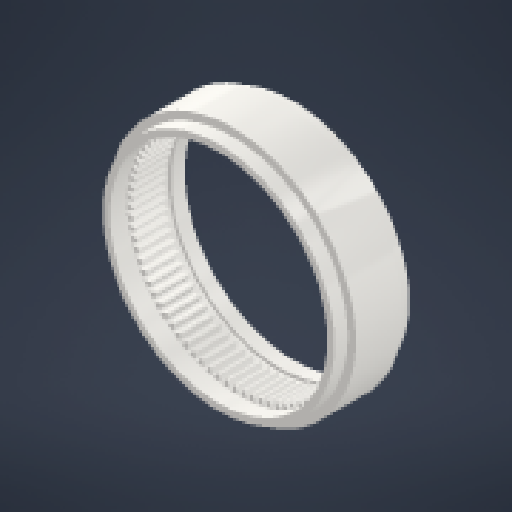
# Autodesk Inventor part: Spur Gear1
Saved by Autodesk Inventor 2024.2 (Build 282272000, 272)
## iProperties
CustomPartVersion: 1
Created: 2026-01-16
Part Number: Spur Gear1
Material: Steel
Document SubType Name: Modeling
Designer: 4aida
Categories: <?xml version="1.0" encoding="UTF-16"?> <MemberInstance><Categories><FamilyTemplate><FamilyTemplateParameter ValueType="xs:double" Id="1" ObjectReferenceKey="da_z" ObjectType="kUserParameterObject"/><FamilyTemplateParameter ValueType="xs:double" Id="2" ObjectReferenceKey="da_b" ObjectType="kUserParameterObject"/><FamilyTemplateParameter ValueType="xs:double" Id="3" ObjectReferenceKey="da_beta" ObjectType="kUserParameterObject"/><FamilyTemplateParameter ValueType="xs:double" Id="4" ObjectReferenceKey="da_da" ObjectType="kUserParameterObject"/><FamilyTemplateParameter ValueType="xs:double" Id="5" ObjectReferenceKey="da_aw" ObjectType="kUserParameterObject"/><FamilyTemplateParameter ValueType="xs:string" Id="6" ObjectReferenceKey="EAIAABAAAACIAQAAAAAAAIAAAAAAAAAA" ObjectType="83910656" SubObjectId="SurfaceGeometry"/></FamilyTemplate><ParamToTemplateMap><ParamToTemplate CategoryParameter="//CategoryParameter[@InternalName='046C89C9-8512-4d59-83FE-43B91F4F132A']" TemplateParameter="1"/><ParamToTemplate CategoryParameter="//CategoryParameter[@InternalName='2552DF32-E462-4b46-AEBF-C6C7768E72AC']" TemplateParameter="2"/><ParamToTemplate CategoryParameter="//CategoryParameter[@InternalName='C9EE641D-15FC-4fae-A226-E94C4372FDD7']" TemplateParameter="3"/><ParamToTemplate><ParamToTemplate CategoryParameter="//CategoryParameter[@InternalName='00B6519A-459B-49c7-AD84-2E56D39A5744']" ConstantValue="0.000000"/></ParamToTemplate><ParamToTemplate><ParamToTemplate CategoryParameter="//CategoryParameter[@InternalName='04B31F0E-C7A6-4894-AA32-9629BEFACF47']" ConstantValue="1.000000"/></ParamToTemplate><ParamToTemplate><ParamToTemplate CategoryParameter="//CategoryParameter[@InternalName='43CBEC2E-7847-49e7-A936-2F7889FCB2D9']" ConstantValue="0.250000"/></ParamToTemplate><ParamToTemplate><ParamToTemplate CategoryParameter="//CategoryParameter[@InternalName='B1EFC894-105D-4ebd-86BF-FA20ED196853']" ConstantValue="0.350000"/></ParamToTemplate><ParamToTemplate><ParamToTemplate CategoryParameter="//CategoryParameter[@InternalName='51175063-3D10-4879-93E8-6246FE8B403D']" ConstantValue="2060000000.000000"/></ParamToTemplate><ParamToTemplate><ParamToTemplate CategoryParameter="//CategoryParameter[@InternalName='A3A52E27-4454-46a9-B0BD-C932399B70AF']" ConstantValue="0.300000"/></ParamToTemplate><ParamToTemplate><ParamToTemplate CategoryParameter="//CategoryParameter[@InternalName='91B76062-C214-41d9-B1B9-14D2AB99603D']" ConstantValue="0.080000"/></ParamToTemplate><ParamToTemplate><ParamToTemplate CategoryParameter="//CategoryParameter[@InternalName='374E806E-8B8A-4dda-A9AA-1039D6500AD2']" ConstantValue="12.500000"/></ParamToTemplate><ParamToTemplate><ParamToTemplate CategoryParameter="//CategoryParameter[@InternalName='2D373A89-B862-43d6-8D0B-0CBF12AB9F6C']" ConstantValue="0.349066"/></ParamToTemplate><ParamToTemplate CategoryParameter="//CategoryParameter[@InternalName='37777632-D6A2-4fac-9D53-DB8ACD95C989']" TemplateParameter="4"/><ParamToTemplate CategoryParameter="//CategoryParameter[@InternalName='FD1017F1-B727-4f7e-9707-0F86F1FF9423']" TemplateParameter="5"/><ParamToTemplate><ParamToTemplate CategoryParameter="//CategoryParameter[@InternalName='9E1B4470-B2D3-4ff1-B813-535BB4CDF51A']" ConstantValue="3520000.000000"/></ParamToTemplate><ParamToTemplate><ParamToTemplate CategoryParameter="//CategoryParameter[@InternalName='F8452263-BFF6-458c-9FB1-07C4B99E95CD']" ConstantValue="11400000.000000"/></ParamToTemplate><ParamToTemplate><ParamToTemplate CategoryParameter="//CategoryParameter[@InternalName='3E3BB259-FD49-497f-8171-6EBC954A3479']" ConstantValue="2.000000"/></ParamToTemplate><ParamToTemplate CategoryParameter="//CategoryParameter[@InternalName='27C3BAF2-7550-4e4b-AE2C-0DB134B7D9B7']" TemplateParameter="6"/></ParamToTemplateMap><Category DisplayName="Gear" InternalName="DC85795E-93AB-48d5-8EEE-5A27447B64BD" Mnemonic="Gear"><CategoryParameter DisplayName="z" InternalName="046C89C9-8512-4d59-83FE-43B91F4F132A" Mnemonic="z"/><CategoryParameter DisplayName="b" InternalName="2552DF32-E462-4b46-AEBF-C6C7768E72AC" Mnemonic="b"/><CategoryParameter DisplayName="||b|" InternalName="C9EE641D-15FC-4fae-A226-E94C4372FDD7" Mnemonic="beta"/><CategoryParameter DisplayName="x" InternalName="00B6519A-459B-49c7-AD84-2E56D39A5744" Mnemonic="x"/><CategoryParameter DisplayName="a*" InternalName="04B31F0E-C7A6-4894-AA32-9629BEFACF47" Mnemonic="a"/><CategoryParameter DisplayName="c*" InternalName="43CBEC2E-7847-49e7-A936-2F7889FCB2D9" Mnemonic="c"/><CategoryParameter DisplayName="r|.f|*" InternalName="B1EFC894-105D-4ebd-86BF-FA20ED196853" Mnemonic="rf"/><CategoryParameter DisplayName="E" InternalName="51175063-3D10-4879-93E8-6246FE8B403D" Mnemonic="E"/><CategoryParameter DisplayName="||m|" InternalName="A3A52E27-4454-46a9-B0BD-C932399B70AF" Mnemonic="mi"/><Category DisplayName="SpurGear" InternalName="26C5A22E-A91E-4dfd-A3B3-23CCAFAE1764" Mnemonic="SpurGear"><CategoryParameter DisplayName="m" InternalName="91B76062-C214-41d9-B1B9-14D2AB99603D" Mnemonic="m"/><CategoryParameter DisplayName="P" InternalName="374E806E-8B8A-4dda-A9AA-1039D6500AD2" Mnemonic="PP"/><CategoryParameter DisplayName="||a|" InternalName="2D373A89-B862-43d6-8D0B-0CBF12AB9F6C" Mnemonic="alpha"/><CategoryParameter DisplayName="d|.a|" InternalName="37777632-D6A2-4fac-9D53-DB8ACD95C989" Mnemonic="da"/><CategoryParameter DisplayName="a|.w|" InternalName="FD1017F1-B727-4f7e-9707-0F86F1FF9423" Mnemonic="aw"/><CategoryParameter DisplayName="||s||.Flim|" InternalName="9E1B4470-B2D3-4ff1-B813-535BB4CDF51A" Mnemonic="sFlim"/><CategoryParameter DisplayName="||s||.Hlim|" InternalName="F8452263-BFF6-458c-9FB1-07C4B99E95CD" Mnemonic="sHlim"/><CategoryParameter DisplayName="type" InternalName="3E3BB259-FD49-497f-8171-6EBC954A3479" Mnemonic="type"/><Category DisplayName="InternalSpurGear" InternalName="7CF704F6-14A9-42f8-93CE-E71DF57C2B55" Mnemonic="InternalSpurGear"><CategoryParameter DisplayName="PitchDiameter" InternalName="27C3BAF2-7550-4e4b-AE2C-0DB134B7D9B7" Mnemonic="IDS_PITCHDIAM"/></Category></Category></Category></Categories></MemberInstance>
Density: 1 g/cm^3
Appearance: Steel
Author: 4aida
Autodesk Inventor part; units mm, degrees
sketch "Sketch1" plane through (0, 0, 0) normal (0, 0, 1) x (1, 0, 0)
  circle A0 centre (0, 0) radius 36.3
  dimension "d0" = 72.6
  constraints: 1 centre point
  measures "d0" diameter of A0
extrude "Extrusion1" add sketch "Sketch1" along normal mid plane 10
ref_plane "Work Plane2" through (0, 0, 0) normal (0, 0, 1) x (1, 0, 0)
sketch "Sketch2" plane through (0, 0, -5) normal (0, 0, -1) x (-1, 0, 0)
  circle A0 centre (0, 0) radius 36.3 projected
  circle A1 centre (0, 0) radius 32
  dimension "d3" = 64
  constraints: 1 centre point, 1 coincident
  measures "d3" diameter of A1
surface extrude "Pitch Diameter" sketch "Sketch2" against normal through all shown no curves A1
ref_plane "Work Plane8" through (0, 0, 0) normal (0.999229, 0.0392598, 0) x (0, 0, 1)
ref_plane "Work Plane9" through (0, 0, 0) normal (1, 0, 0) x (0, 1, 0)
spur gear teeth "Spur Gear" teeth 80 pitch diameter 64 tip diameter 62.4 root diameter 66 face width 10 start plane through (0, 0, -5) normal (0, 0, -1) x (-1, 0, 0)
sketch "Sketch3" plane through (0, 0, 5) normal (0, 0, 1) x (1, 0, 0)
  arc A0 (2.912, -32.8713) -> (3.3628, -31.0182) centre (-7.2848, -29.4092) ccw projected
  arc A1 (2.2661, -32.9221) -> (2.912, -32.8713) centre (0, 0) ccw projected
  arc A2 (1.5309, -31.1624) -> (2.2661, -32.9221) centre (11.7957, -27.9075) ccw projected
  arc A3 (0.9188, -31.1865) -> (1.5309, -31.1624) centre (0, 0) ccw projected
  arc A4 (0.324, -32.9984) -> (0.9188, -31.1865) centre (-9.5697, -28.747) ccw projected
  arc A5 (-0.324, -32.9984) -> (0.324, -32.9984) centre (0, 0) ccw projected
  arc A6 (-0.9188, -31.1865) -> (-0.324, -32.9984) centre (9.5697, -28.747) ccw projected
  arc A7 (-1.5309, -31.1624) -> (-0.9188, -31.1865) centre (0, 0) ccw projected
  arc A8 (-2.2661, -32.9221) -> (-1.5309, -31.1624) centre (-11.7957, -27.9075) ccw projected
  arc A9 (-2.912, -32.8713) -> (-2.2661, -32.9221) centre (0, 0) ccw projected
  arc A10 (-3.3628, -31.0182) -> (-2.912, -32.8713) centre (7.2848, -29.4092) ccw projected
  arc A11 (-3.9712, -30.9462) -> (-3.3628, -31.0182) centre (0, 0) ccw projected
  arc A12 (-4.8421, -32.6428) -> (-3.9712, -30.9462) centre (-13.9489, -26.896) ccw projected
  arc A13 (-5.4821, -32.5415) -> (-4.8421, -32.6428) centre (0, 0) ccw projected
  arc A14 (-5.7861, -30.6588) -> (-5.4821, -32.5415) centre (4.9549, -29.8901) ccw projected
  arc A15 (-6.3869, -30.5393) -> (-5.7861, -30.6588) centre (0, 0) ccw projected
  arc A16 (-7.3883, -32.1623) -> (-6.3869, -30.5393) centre (-16.0162, -25.7187) ccw projected
  arc A17 (-8.0183, -32.011) -> (-7.3883, -32.1623) centre (0, 0) ccw projected
  arc A18 (-8.1737, -30.1103) -> (-8.0183, -32.011) centre (2.5945, -30.1867) ccw projected
  arc A19 (-8.7633, -29.944) -> (-8.1737, -30.1103) centre (0, 0) ccw projected
  arc A20 (-9.889, -31.4835) -> (-8.7633, -29.944) centre (-17.9847, -24.3828) ccw projected
  arc A21 (-10.5052, -31.2832) -> (-9.889, -31.4835) centre (0, 0) ccw projected
  arc A22 (-10.511, -29.3762) -> (-10.5052, -31.2832) centre (0.218, -30.2972) ccw projected
  arc A23 (-11.0857, -29.1641) -> (-10.511, -29.3762) centre (0, 0) ccw projected
  arc A24 (-12.3286, -30.6105) -> (-11.0857, -29.1641) centre (-19.8423, -22.8966) ccw projected
  arc A25 (-12.9273, -30.3626) -> (-12.3286, -30.6105) centre (0, 0) ccw projected
  arc A26 (-12.7834, -28.4609) -> (-12.9273, -30.3626) centre (-2.1597, -30.2209) ccw projected
  arc A27 (-13.3397, -28.2045) -> (-12.7834, -28.4609) centre (0, 0) ccw projected
  arc A28 (-14.6923, -29.5489) -> (-13.3397, -28.2045) centre (-21.5775, -21.2692) ccw projected
  arc A29 (-15.2696, -29.2547) -> (-14.6923, -29.5489) centre (0, 0) ccw projected
  arc A30 (-14.977, -27.3702) -> (-15.2696, -29.2547) centre (-4.5242, -29.9583) ccw projected
  arc A31 (-15.5115, -27.0709) -> (-14.977, -27.3702) centre (0, 0) ccw projected
  arc A32 (-16.9654, -28.305) -> (-15.5115, -27.0709) centre (-23.1798, -19.5107) ccw projected
  arc A33 (-17.5179, -27.9665) -> (-16.9654, -28.305) centre (0, 0) ccw projected
  arc A34 (-17.0783, -26.1108) -> (-17.5179, -27.9665) centre (-6.8607, -29.511) ccw projected
  arc A35 (-17.5876, -25.7704) -> (-17.0783, -26.1108) centre (0, 0) ccw projected
  arc A36 (-19.1339, -26.8867) -> (-17.5876, -25.7704) centre (-24.6391, -17.6318) ccw projected
  arc A37 (-19.6581, -26.5058) -> (-19.1339, -26.8867) centre (0, 0) ccw projected
  arc A38 (-19.0743, -24.6903) -> (-19.6581, -26.5058) centre (-9.155, -28.8817) ccw projected
  arc A39 (-19.5553, -24.3111) -> (-19.0743, -24.6903) centre (0, 0) ccw projected
  arc A40 (-21.1844, -25.3026) -> (-19.5553, -24.3111) centre (-25.9465, -15.6443) ccw projected
  arc A41 (-21.6771, -24.8818) -> (-21.1844, -25.3026) centre (0, 0) ccw projected
  arc A42 (-20.9526, -23.1177) -> (-21.6771, -24.8818) centre (-11.3928, -28.0744) ccw projected
  arc A43 (-21.4025, -22.7018) -> (-20.9526, -23.1177) centre (0, 0) ccw projected
  arc A44 (-23.1043, -23.5625) -> (-21.4025, -22.7018) centre (-27.094, -13.5604) ccw projected
  arc A45 (-23.5625, -23.1043) -> (-23.1043, -23.5625) centre (0, 0) ccw projected
  arc A46 (-22.7018, -21.4025) -> (-23.5625, -23.1043) centre (-13.5604, -27.094) ccw projected
  arc A47 (-23.1177, -20.9526) -> (-22.7018, -21.4025) centre (0, 0) ccw projected
  arc A48 (-24.8818, -21.6771) -> (-23.1177, -20.9526) centre (-28.0744, -11.3928) ccw projected
  arc A49 (-25.3026, -21.1844) -> (-24.8818, -21.6771) centre (0, 0) ccw projected
  arc A50 (-24.3111, -19.5553) -> (-25.3026, -21.1844) centre (-15.6443, -25.9465) ccw projected
  arc A51 (-24.6903, -19.0743) -> (-24.3111, -19.5553) centre (0, 0) ccw projected
  arc A52 (-26.5058, -19.6581) -> (-24.6903, -19.0743) centre (-28.8817, -9.155) ccw projected
  arc A53 (-26.8867, -19.1339) -> (-26.5058, -19.6581) centre (0, 0) ccw projected
  arc A54 (-25.7704, -17.5876) -> (-26.8867, -19.1339) centre (-17.6318, -24.6391) ccw projected
  arc A55 (-26.1108, -17.0783) -> (-25.7704, -17.5876) centre (0, 0) ccw projected
  arc A56 (-27.9665, -17.5179) -> (-26.1108, -17.0783) centre (-29.511, -6.8607) ccw projected
  arc A57 (-28.305, -16.9654) -> (-27.9665, -17.5179) centre (0, 0) ccw projected
  arc A58 (-27.0709, -15.5115) -> (-28.305, -16.9654) centre (-19.5107, -23.1798) ccw projected
  arc A59 (-27.3702, -14.977) -> (-27.0709, -15.5115) centre (0, 0) ccw projected
  arc A60 (-29.2547, -15.2696) -> (-27.3702, -14.977) centre (-29.9583, -4.5242) ccw projected
  arc A61 (-29.5489, -14.6923) -> (-29.2547, -15.2696) centre (0, 0) ccw projected
  arc A62 (-28.2045, -13.3397) -> (-29.5489, -14.6923) centre (-21.2692, -21.5775) ccw projected
  arc A63 (-28.4609, -12.7834) -> (-28.2045, -13.3397) centre (0, 0) ccw projected
  arc A64 (-30.3626, -12.9273) -> (-28.4609, -12.7834) centre (-30.2209, -2.1597) ccw projected
  arc A65 (-30.6105, -12.3286) -> (-30.3626, -12.9273) centre (0, 0) ccw projected
  arc A66 (-29.1641, -11.0857) -> (-30.6105, -12.3286) centre (-22.8966, -19.8423) ccw projected
  arc A67 (-29.3762, -10.511) -> (-29.1641, -11.0857) centre (0, 0) ccw projected
  arc A68 (-31.2832, -10.5052) -> (-29.3762, -10.511) centre (-30.2972, 0.218) ccw projected
  arc A69 (-31.4835, -9.889) -> (-31.2832, -10.5052) centre (0, 0) ccw projected
  arc A70 (-29.944, -8.7633) -> (-31.4835, -9.889) centre (-24.3828, -17.9847) ccw projected
  arc A71 (-30.1103, -8.1737) -> (-29.944, -8.7633) centre (0, 0) ccw projected
  arc A72 (-32.011, -8.0183) -> (-30.1103, -8.1737) centre (-30.1867, 2.5945) ccw projected
  arc A73 (-32.1623, -7.3883) -> (-32.011, -8.0183) centre (0, 0) ccw projected
  arc A74 (-30.5393, -6.3869) -> (-32.1623, -7.3883) centre (-25.7187, -16.0162) ccw projected
  arc A75 (-30.6588, -5.7861) -> (-30.5393, -6.3869) centre (0, 0) ccw projected
  arc A76 (-32.5415, -5.4821) -> (-30.6588, -5.7861) centre (-29.8901, 4.9549) ccw projected
  arc A77 (-32.6428, -4.8421) -> (-32.5415, -5.4821) centre (0, 0) ccw projected
  arc A78 (-30.9462, -3.9712) -> (-32.6428, -4.8421) centre (-26.896, -13.9489) ccw projected
  arc A79 (-31.0182, -3.3628) -> (-30.9462, -3.9712) centre (0, 0) ccw projected
  arc A80 (-32.8713, -2.912) -> (-31.0182, -3.3628) centre (-29.4092, 7.2848) ccw projected
  arc A81 (-32.9221, -2.2661) -> (-32.8713, -2.912) centre (0, 0) ccw projected
  arc A82 (-31.1624, -1.5309) -> (-32.9221, -2.2661) centre (-27.9075, -11.7957) ccw projected
  arc A83 (-31.1865, -0.9188) -> (-31.1624, -1.5309) centre (0, 0) ccw projected
  arc A84 (-32.9984, -0.324) -> (-31.1865, -0.9188) centre (-28.747, 9.5697) ccw projected
  arc A85 (-32.9984, 0.324) -> (-32.9984, -0.324) centre (0, 0) ccw projected
  arc A86 (-31.1865, 0.9188) -> (-32.9984, 0.324) centre (-28.747, -9.5697) ccw projected
  arc A87 (-31.1624, 1.5309) -> (-31.1865, 0.9188) centre (0, 0) ccw projected
  arc A88 (-32.9221, 2.2661) -> (-31.1624, 1.5309) centre (-27.9075, 11.7957) ccw projected
  arc A89 (-32.8713, 2.912) -> (-32.9221, 2.2661) centre (0, 0) ccw projected
  arc A90 (-31.0182, 3.3628) -> (-32.8713, 2.912) centre (-29.4092, -7.2848) ccw projected
  arc A91 (-30.9462, 3.9712) -> (-31.0182, 3.3628) centre (0, 0) ccw projected
  arc A92 (-32.6428, 4.8421) -> (-30.9462, 3.9712) centre (-26.896, 13.9489) ccw projected
  arc A93 (-32.5415, 5.4821) -> (-32.6428, 4.8421) centre (0, 0) ccw projected
  arc A94 (-30.6588, 5.7861) -> (-32.5415, 5.4821) centre (-29.8901, -4.9549) ccw projected
  arc A95 (-30.5393, 6.3869) -> (-30.6588, 5.7861) centre (0, 0) ccw projected
  arc A96 (-32.1623, 7.3883) -> (-30.5393, 6.3869) centre (-25.7187, 16.0162) ccw projected
  arc A97 (-32.011, 8.0183) -> (-32.1623, 7.3883) centre (0, 0) ccw projected
  arc A98 (-30.1103, 8.1737) -> (-32.011, 8.0183) centre (-30.1867, -2.5945) ccw projected
  arc A99 (-29.944, 8.7633) -> (-30.1103, 8.1737) centre (0, 0) ccw projected
  arc A100 (-31.4835, 9.889) -> (-29.944, 8.7633) centre (-24.3828, 17.9847) ccw projected
  arc A101 (-31.2832, 10.5052) -> (-31.4835, 9.889) centre (0, 0) ccw projected
  arc A102 (-29.3762, 10.511) -> (-31.2832, 10.5052) centre (-30.2972, -0.218) ccw projected
  arc A103 (-29.1641, 11.0857) -> (-29.3762, 10.511) centre (0, 0) ccw projected
  arc A104 (-30.6105, 12.3286) -> (-29.1641, 11.0857) centre (-22.8966, 19.8423) ccw projected
  arc A105 (-30.3626, 12.9273) -> (-30.6105, 12.3286) centre (0, 0) ccw projected
  arc A106 (-28.4609, 12.7834) -> (-30.3626, 12.9273) centre (-30.2209, 2.1597) ccw projected
  arc A107 (-28.2045, 13.3397) -> (-28.4609, 12.7834) centre (0, 0) ccw projected
  arc A108 (-29.5489, 14.6923) -> (-28.2045, 13.3397) centre (-21.2692, 21.5775) ccw projected
  arc A109 (-29.2547, 15.2696) -> (-29.5489, 14.6923) centre (0, 0) ccw projected
  arc A110 (-27.3702, 14.977) -> (-29.2547, 15.2696) centre (-29.9583, 4.5242) ccw projected
  arc A111 (-27.0709, 15.5115) -> (-27.3702, 14.977) centre (0, 0) ccw projected
  arc A112 (-28.305, 16.9654) -> (-27.0709, 15.5115) centre (-19.5107, 23.1798) ccw projected
  arc A113 (-27.9665, 17.5179) -> (-28.305, 16.9654) centre (0, 0) ccw projected
  arc A114 (-26.1108, 17.0783) -> (-27.9665, 17.5179) centre (-29.511, 6.8607) ccw projected
  arc A115 (-25.7704, 17.5876) -> (-26.1108, 17.0783) centre (0, 0) ccw projected
  arc A116 (-26.8867, 19.1339) -> (-25.7704, 17.5876) centre (-17.6318, 24.6391) ccw projected
  arc A117 (-26.5058, 19.6581) -> (-26.8867, 19.1339) centre (0, 0) ccw projected
  arc A118 (-24.6903, 19.0743) -> (-26.5058, 19.6581) centre (-28.8817, 9.155) ccw projected
  arc A119 (-24.3111, 19.5553) -> (-24.6903, 19.0743) centre (0, 0) ccw projected
  arc A120 (-25.3026, 21.1844) -> (-24.3111, 19.5553) centre (-15.6443, 25.9465) ccw projected
  arc A121 (-24.8818, 21.6771) -> (-25.3026, 21.1844) centre (0, 0) ccw projected
  arc A122 (-23.1177, 20.9526) -> (-24.8818, 21.6771) centre (-28.0744, 11.3928) ccw projected
  arc A123 (-22.7018, 21.4025) -> (-23.1177, 20.9526) centre (0, 0) ccw projected
  arc A124 (-23.5625, 23.1043) -> (-22.7018, 21.4025) centre (-13.5604, 27.094) ccw projected
  arc A125 (-23.1043, 23.5625) -> (-23.5625, 23.1043) centre (0, 0) ccw projected
  arc A126 (-21.4025, 22.7018) -> (-23.1043, 23.5625) centre (-27.094, 13.5604) ccw projected
  arc A127 (-20.9526, 23.1177) -> (-21.4025, 22.7018) centre (0, 0) ccw projected
  arc A128 (-21.6771, 24.8818) -> (-20.9526, 23.1177) centre (-11.3928, 28.0744) ccw projected
  arc A129 (-21.1844, 25.3026) -> (-21.6771, 24.8818) centre (0, 0) ccw projected
  arc A130 (-19.5553, 24.3111) -> (-21.1844, 25.3026) centre (-25.9465, 15.6443) ccw projected
  arc A131 (-19.0743, 24.6903) -> (-19.5553, 24.3111) centre (0, 0) ccw projected
  arc A132 (-19.6581, 26.5058) -> (-19.0743, 24.6903) centre (-9.155, 28.8817) ccw projected
  arc A133 (-19.1339, 26.8867) -> (-19.6581, 26.5058) centre (0, 0) ccw projected
  arc A134 (-17.5876, 25.7704) -> (-19.1339, 26.8867) centre (-24.6391, 17.6318) ccw projected
  arc A135 (-17.0783, 26.1108) -> (-17.5876, 25.7704) centre (0, 0) ccw projected
  arc A136 (-17.5179, 27.9665) -> (-17.0783, 26.1108) centre (-6.8607, 29.511) ccw projected
  arc A137 (-16.9654, 28.305) -> (-17.5179, 27.9665) centre (0, 0) ccw projected
  arc A138 (-15.5115, 27.0709) -> (-16.9654, 28.305) centre (-23.1798, 19.5107) ccw projected
  arc A139 (-14.977, 27.3702) -> (-15.5115, 27.0709) centre (0, 0) ccw projected
  arc A140 (-15.2696, 29.2547) -> (-14.977, 27.3702) centre (-4.5242, 29.9583) ccw projected
  arc A141 (-14.6923, 29.5489) -> (-15.2696, 29.2547) centre (0, 0) ccw projected
  arc A142 (-13.3397, 28.2045) -> (-14.6923, 29.5489) centre (-21.5775, 21.2692) ccw projected
  arc A143 (-12.7834, 28.4609) -> (-13.3397, 28.2045) centre (0, 0) ccw projected
  arc A144 (-12.9273, 30.3626) -> (-12.7834, 28.4609) centre (-2.1597, 30.2209) ccw projected
  arc A145 (-12.3286, 30.6105) -> (-12.9273, 30.3626) centre (0, 0) ccw projected
  arc A146 (-11.0857, 29.1641) -> (-12.3286, 30.6105) centre (-19.8423, 22.8966) ccw projected
  arc A147 (-10.511, 29.3762) -> (-11.0857, 29.1641) centre (0, 0) ccw projected
  arc A148 (-10.5052, 31.2832) -> (-10.511, 29.3762) centre (0.218, 30.2972) ccw projected
  arc A149 (-9.889, 31.4835) -> (-10.5052, 31.2832) centre (0, 0) ccw projected
  arc A150 (-8.7633, 29.944) -> (-9.889, 31.4835) centre (-17.9847, 24.3828) ccw projected
  arc A151 (-8.1737, 30.1103) -> (-8.7633, 29.944) centre (0, 0) ccw projected
  arc A152 (-8.0183, 32.011) -> (-8.1737, 30.1103) centre (2.5945, 30.1867) ccw projected
  arc A153 (-7.3883, 32.1623) -> (-8.0183, 32.011) centre (0, 0) ccw projected
  arc A154 (-6.3869, 30.5393) -> (-7.3883, 32.1623) centre (-16.0162, 25.7187) ccw projected
  arc A155 (-5.7861, 30.6588) -> (-6.3869, 30.5393) centre (0, 0) ccw projected
  arc A156 (-5.4821, 32.5415) -> (-5.7861, 30.6588) centre (4.9549, 29.8901) ccw projected
  arc A157 (-4.8421, 32.6428) -> (-5.4821, 32.5415) centre (0, 0) ccw projected
  arc A158 (-3.9712, 30.9462) -> (-4.8421, 32.6428) centre (-13.9489, 26.896) ccw projected
  arc A159 (-3.3628, 31.0182) -> (-3.9712, 30.9462) centre (0, 0) ccw projected
  arc A160 (-2.912, 32.8713) -> (-3.3628, 31.0182) centre (7.2848, 29.4092) ccw projected
  arc A161 (-2.2661, 32.9221) -> (-2.912, 32.8713) centre (0, 0) ccw projected
  arc A162 (-1.5309, 31.1624) -> (-2.2661, 32.9221) centre (-11.7957, 27.9075) ccw projected
  arc A163 (-0.9188, 31.1865) -> (-1.5309, 31.1624) centre (0, 0) ccw projected
  arc A164 (-0.324, 32.9984) -> (-0.9188, 31.1865) centre (9.5697, 28.747) ccw projected
  arc A165 (0.324, 32.9984) -> (-0.324, 32.9984) centre (0, 0) ccw projected
  arc A166 (0.9188, 31.1865) -> (0.324, 32.9984) centre (-9.5697, 28.747) ccw projected
  arc A167 (1.5309, 31.1624) -> (0.9188, 31.1865) centre (0, 0) ccw projected
  arc A168 (2.2661, 32.9221) -> (1.5309, 31.1624) centre (11.7957, 27.9075) ccw projected
  arc A169 (2.912, 32.8713) -> (2.2661, 32.9221) centre (0, 0) ccw projected
  arc A170 (3.3628, 31.0182) -> (2.912, 32.8713) centre (-7.2848, 29.4092) ccw projected
  arc A171 (3.9712, 30.9462) -> (3.3628, 31.0182) centre (0, 0) ccw projected
  arc A172 (4.8421, 32.6428) -> (3.9712, 30.9462) centre (13.9489, 26.896) ccw projected
  arc A173 (5.4821, 32.5415) -> (4.8421, 32.6428) centre (0, 0) ccw projected
  arc A174 (5.7861, 30.6588) -> (5.4821, 32.5415) centre (-4.9549, 29.8901) ccw projected
  arc A175 (6.3869, 30.5393) -> (5.7861, 30.6588) centre (0, 0) ccw projected
  arc A176 (7.3883, 32.1623) -> (6.3869, 30.5393) centre (16.0162, 25.7187) ccw projected
  arc A177 (8.0183, 32.011) -> (7.3883, 32.1623) centre (0, 0) ccw projected
  arc A178 (8.1737, 30.1103) -> (8.0183, 32.011) centre (-2.5945, 30.1867) ccw projected
  arc A179 (8.7633, 29.944) -> (8.1737, 30.1103) centre (0, 0) ccw projected
  arc A180 (9.889, 31.4835) -> (8.7633, 29.944) centre (17.9847, 24.3828) ccw projected
  arc A181 (10.5052, 31.2832) -> (9.889, 31.4835) centre (0, 0) ccw projected
  arc A182 (10.511, 29.3762) -> (10.5052, 31.2832) centre (-0.218, 30.2972) ccw projected
  arc A183 (11.0857, 29.1641) -> (10.511, 29.3762) centre (0, 0) ccw projected
  arc A184 (12.3286, 30.6105) -> (11.0857, 29.1641) centre (19.8423, 22.8966) ccw projected
  arc A185 (12.9273, 30.3626) -> (12.3286, 30.6105) centre (0, 0) ccw projected
  arc A186 (12.7834, 28.4609) -> (12.9273, 30.3626) centre (2.1597, 30.2209) ccw projected
  arc A187 (13.3397, 28.2045) -> (12.7834, 28.4609) centre (0, 0) ccw projected
  arc A188 (14.6923, 29.5489) -> (13.3397, 28.2045) centre (21.5775, 21.2692) ccw projected
  arc A189 (15.2696, 29.2547) -> (14.6923, 29.5489) centre (0, 0) ccw projected
  arc A190 (14.977, 27.3702) -> (15.2696, 29.2547) centre (4.5242, 29.9583) ccw projected
  arc A191 (15.5115, 27.0709) -> (14.977, 27.3702) centre (0, 0) ccw projected
  arc A192 (16.9654, 28.305) -> (15.5115, 27.0709) centre (23.1798, 19.5107) ccw projected
  arc A193 (17.5179, 27.9665) -> (16.9654, 28.305) centre (0, 0) ccw projected
  arc A194 (17.0783, 26.1108) -> (17.5179, 27.9665) centre (6.8607, 29.511) ccw projected
  arc A195 (17.5876, 25.7704) -> (17.0783, 26.1108) centre (0, 0) ccw projected
  arc A196 (19.1339, 26.8867) -> (17.5876, 25.7704) centre (24.6391, 17.6318) ccw projected
  arc A197 (19.6581, 26.5058) -> (19.1339, 26.8867) centre (0, 0) ccw projected
  arc A198 (19.0743, 24.6903) -> (19.6581, 26.5058) centre (9.155, 28.8817) ccw projected
  arc A199 (19.5553, 24.3111) -> (19.0743, 24.6903) centre (0, 0) ccw projected
  arc A200 (21.1844, 25.3026) -> (19.5553, 24.3111) centre (25.9465, 15.6443) ccw projected
  arc A201 (21.6771, 24.8818) -> (21.1844, 25.3026) centre (0, 0) ccw projected
  arc A202 (20.9526, 23.1177) -> (21.6771, 24.8818) centre (11.3928, 28.0744) ccw projected
  arc A203 (21.4025, 22.7018) -> (20.9526, 23.1177) centre (0, 0) ccw projected
  arc A204 (23.1043, 23.5625) -> (21.4025, 22.7018) centre (27.094, 13.5604) ccw projected
  arc A205 (23.5625, 23.1043) -> (23.1043, 23.5625) centre (0, 0) ccw projected
  arc A206 (22.7018, 21.4025) -> (23.5625, 23.1043) centre (13.5604, 27.094) ccw projected
  arc A207 (23.1177, 20.9526) -> (22.7018, 21.4025) centre (0, 0) ccw projected
  arc A208 (24.8818, 21.6771) -> (23.1177, 20.9526) centre (28.0744, 11.3928) ccw projected
  arc A209 (25.3026, 21.1844) -> (24.8818, 21.6771) centre (0, 0) ccw projected
  arc A210 (24.3111, 19.5553) -> (25.3026, 21.1844) centre (15.6443, 25.9465) ccw projected
  arc A211 (24.6903, 19.0743) -> (24.3111, 19.5553) centre (0, 0) ccw projected
  arc A212 (26.5058, 19.6581) -> (24.6903, 19.0743) centre (28.8817, 9.155) ccw projected
  arc A213 (26.8867, 19.1339) -> (26.5058, 19.6581) centre (0, 0) ccw projected
  arc A214 (25.7704, 17.5876) -> (26.8867, 19.1339) centre (17.6318, 24.6391) ccw projected
  arc A215 (26.1108, 17.0783) -> (25.7704, 17.5876) centre (0, 0) ccw projected
  arc A216 (27.9665, 17.5179) -> (26.1108, 17.0783) centre (29.511, 6.8607) ccw projected
  arc A217 (28.305, 16.9654) -> (27.9665, 17.5179) centre (0, 0) ccw projected
  arc A218 (27.0709, 15.5115) -> (28.305, 16.9654) centre (19.5107, 23.1798) ccw projected
  arc A219 (27.3702, 14.977) -> (27.0709, 15.5115) centre (0, 0) ccw projected
  arc A220 (29.2547, 15.2696) -> (27.3702, 14.977) centre (29.9583, 4.5242) ccw projected
  arc A221 (29.5489, 14.6923) -> (29.2547, 15.2696) centre (0, 0) ccw projected
  arc A222 (28.2045, 13.3397) -> (29.5489, 14.6923) centre (21.2692, 21.5775) ccw projected
  arc A223 (28.4609, 12.7834) -> (28.2045, 13.3397) centre (0, 0) ccw projected
  arc A224 (30.3626, 12.9273) -> (28.4609, 12.7834) centre (30.2209, 2.1597) ccw projected
  arc A225 (30.6105, 12.3286) -> (30.3626, 12.9273) centre (0, 0) ccw projected
  arc A226 (29.1641, 11.0857) -> (30.6105, 12.3286) centre (22.8966, 19.8423) ccw projected
  arc A227 (29.3762, 10.511) -> (29.1641, 11.0857) centre (0, 0) ccw projected
  arc A228 (31.2832, 10.5052) -> (29.3762, 10.511) centre (30.2972, -0.218) ccw projected
  arc A229 (31.4835, 9.889) -> (31.2832, 10.5052) centre (0, 0) ccw projected
  arc A230 (29.944, 8.7633) -> (31.4835, 9.889) centre (24.3828, 17.9847) ccw projected
  arc A231 (30.1103, 8.1737) -> (29.944, 8.7633) centre (0, 0) ccw projected
  arc A232 (32.011, 8.0183) -> (30.1103, 8.1737) centre (30.1867, -2.5945) ccw projected
  arc A233 (32.1623, 7.3883) -> (32.011, 8.0183) centre (0, 0) ccw projected
  arc A234 (30.5393, 6.3869) -> (32.1623, 7.3883) centre (25.7187, 16.0162) ccw projected
  arc A235 (30.6588, 5.7861) -> (30.5393, 6.3869) centre (0, 0) ccw projected
  arc A236 (32.5415, 5.4821) -> (30.6588, 5.7861) centre (29.8901, -4.9549) ccw projected
  arc A237 (32.6428, 4.8421) -> (32.5415, 5.4821) centre (0, 0) ccw projected
  arc A238 (30.9462, 3.9712) -> (32.6428, 4.8421) centre (26.896, 13.9489) ccw projected
  arc A239 (31.0182, 3.3628) -> (30.9462, 3.9712) centre (0, 0) ccw projected
  arc A240 (32.8713, 2.912) -> (31.0182, 3.3628) centre (29.4092, -7.2848) ccw projected
  arc A241 (32.9221, 2.2661) -> (32.8713, 2.912) centre (0, 0) ccw projected
  arc A242 (31.1624, 1.5309) -> (32.9221, 2.2661) centre (27.9075, 11.7957) ccw projected
  arc A243 (31.1865, 0.9188) -> (31.1624, 1.5309) centre (0, 0) ccw projected
  arc A244 (32.9984, 0.324) -> (31.1865, 0.9188) centre (28.747, -9.5697) ccw projected
  arc A245 (32.9984, -0.324) -> (32.9984, 0.324) centre (0, 0) ccw projected
  arc A246 (31.1865, -0.9188) -> (32.9984, -0.324) centre (28.747, 9.5697) ccw projected
  arc A247 (31.1624, -1.5309) -> (31.1865, -0.9188) centre (0, 0) ccw projected
  arc A248 (32.9221, -2.2661) -> (31.1624, -1.5309) centre (27.9075, -11.7957) ccw projected
  arc A249 (32.8713, -2.912) -> (32.9221, -2.2661) centre (0, 0) ccw projected
  arc A250 (31.0182, -3.3628) -> (32.8713, -2.912) centre (29.4092, 7.2848) ccw projected
  arc A251 (30.9462, -3.9712) -> (31.0182, -3.3628) centre (0, 0) ccw projected
  arc A252 (32.6428, -4.8421) -> (30.9462, -3.9712) centre (26.896, -13.9489) ccw projected
  arc A253 (32.5415, -5.4821) -> (32.6428, -4.8421) centre (0, 0) ccw projected
  arc A254 (30.6588, -5.7861) -> (32.5415, -5.4821) centre (29.8901, 4.9549) ccw projected
  arc A255 (30.5393, -6.3869) -> (30.6588, -5.7861) centre (0, 0) ccw projected
  arc A256 (32.1623, -7.3883) -> (30.5393, -6.3869) centre (25.7187, -16.0162) ccw projected
  arc A257 (32.011, -8.0183) -> (32.1623, -7.3883) centre (0, 0) ccw projected
  arc A258 (30.1103, -8.1737) -> (32.011, -8.0183) centre (30.1867, 2.5945) ccw projected
  arc A259 (29.944, -8.7633) -> (30.1103, -8.1737) centre (0, 0) ccw projected
  arc A260 (31.4835, -9.889) -> (29.944, -8.7633) centre (24.3828, -17.9847) ccw projected
  arc A261 (31.2832, -10.5052) -> (31.4835, -9.889) centre (0, 0) ccw projected
  arc A262 (29.3762, -10.511) -> (31.2832, -10.5052) centre (30.2972, 0.218) ccw projected
  arc A263 (29.1641, -11.0857) -> (29.3762, -10.511) centre (0, 0) ccw projected
  arc A264 (30.6105, -12.3286) -> (29.1641, -11.0857) centre (22.8966, -19.8423) ccw projected
  arc A265 (30.3626, -12.9273) -> (30.6105, -12.3286) centre (0, 0) ccw projected
  arc A266 (28.4609, -12.7834) -> (30.3626, -12.9273) centre (30.2209, -2.1597) ccw projected
  arc A267 (28.2045, -13.3397) -> (28.4609, -12.7834) centre (0, 0) ccw projected
  arc A268 (29.5489, -14.6923) -> (28.2045, -13.3397) centre (21.2692, -21.5775) ccw projected
  arc A269 (29.2547, -15.2696) -> (29.5489, -14.6923) centre (0, 0) ccw projected
  arc A270 (27.3702, -14.977) -> (29.2547, -15.2696) centre (29.9583, -4.5242) ccw projected
  arc A271 (27.0709, -15.5115) -> (27.3702, -14.977) centre (0, 0) ccw projected
  arc A272 (28.305, -16.9654) -> (27.0709, -15.5115) centre (19.5107, -23.1798) ccw projected
  arc A273 (27.9665, -17.5179) -> (28.305, -16.9654) centre (0, 0) ccw projected
  arc A274 (26.1108, -17.0783) -> (27.9665, -17.5179) centre (29.511, -6.8607) ccw projected
  arc A275 (25.7704, -17.5876) -> (26.1108, -17.0783) centre (0, 0) ccw projected
  arc A276 (26.8867, -19.1339) -> (25.7704, -17.5876) centre (17.6318, -24.6391) ccw projected
  arc A277 (26.5058, -19.6581) -> (26.8867, -19.1339) centre (0, 0) ccw projected
  arc A278 (24.6903, -19.0743) -> (26.5058, -19.6581) centre (28.8817, -9.155) ccw projected
  arc A279 (24.3111, -19.5553) -> (24.6903, -19.0743) centre (0, 0) ccw projected
  arc A280 (25.3026, -21.1844) -> (24.3111, -19.5553) centre (15.6443, -25.9465) ccw projected
  arc A281 (24.8818, -21.6771) -> (25.3026, -21.1844) centre (0, 0) ccw projected
  arc A282 (23.1177, -20.9526) -> (24.8818, -21.6771) centre (28.0744, -11.3928) ccw projected
  arc A283 (22.7018, -21.4025) -> (23.1177, -20.9526) centre (0, 0) ccw projected
  arc A284 (23.5625, -23.1043) -> (22.7018, -21.4025) centre (13.5604, -27.094) ccw projected
  arc A285 (23.1043, -23.5625) -> (23.5625, -23.1043) centre (0, 0) ccw projected
  arc A286 (21.4025, -22.7018) -> (23.1043, -23.5625) centre (27.094, -13.5604) ccw projected
  arc A287 (20.9526, -23.1177) -> (21.4025, -22.7018) centre (0, 0) ccw projected
  arc A288 (21.6771, -24.8818) -> (20.9526, -23.1177) centre (11.3928, -28.0744) ccw projected
  arc A289 (21.1844, -25.3026) -> (21.6771, -24.8818) centre (0, 0) ccw projected
  arc A290 (19.5553, -24.3111) -> (21.1844, -25.3026) centre (25.9465, -15.6443) ccw projected
  arc A291 (19.0743, -24.6903) -> (19.5553, -24.3111) centre (0, 0) ccw projected
  arc A292 (19.6581, -26.5058) -> (19.0743, -24.6903) centre (9.155, -28.8817) ccw projected
  arc A293 (19.1339, -26.8867) -> (19.6581, -26.5058) centre (0, 0) ccw projected
  arc A294 (17.5876, -25.7704) -> (19.1339, -26.8867) centre (24.6391, -17.6318) ccw projected
  arc A295 (17.0783, -26.1108) -> (17.5876, -25.7704) centre (0, 0) ccw projected
  arc A296 (17.5179, -27.9665) -> (17.0783, -26.1108) centre (6.8607, -29.511) ccw projected
  arc A297 (16.9654, -28.305) -> (17.5179, -27.9665) centre (0, 0) ccw projected
  arc A298 (15.5115, -27.0709) -> (16.9654, -28.305) centre (23.1798, -19.5107) ccw projected
  arc A299 (14.977, -27.3702) -> (15.5115, -27.0709) centre (0, 0) ccw projected
  arc A300 (15.2696, -29.2547) -> (14.977, -27.3702) centre (4.5242, -29.9583) ccw projected
  arc A301 (14.6923, -29.5489) -> (15.2696, -29.2547) centre (0, 0) ccw projected
  arc A302 (13.3397, -28.2045) -> (14.6923, -29.5489) centre (21.5775, -21.2692) ccw projected
  arc A303 (12.7834, -28.4609) -> (13.3397, -28.2045) centre (0, 0) ccw projected
  arc A304 (12.9273, -30.3626) -> (12.7834, -28.4609) centre (2.1597, -30.2209) ccw projected
  arc A305 (12.3286, -30.6105) -> (12.9273, -30.3626) centre (0, 0) ccw projected
  arc A306 (11.0857, -29.1641) -> (12.3286, -30.6105) centre (19.8423, -22.8966) ccw projected
  arc A307 (10.511, -29.3762) -> (11.0857, -29.1641) centre (0, 0) ccw projected
  arc A308 (10.5052, -31.2832) -> (10.511, -29.3762) centre (-0.218, -30.2972) ccw projected
  arc A309 (9.889, -31.4835) -> (10.5052, -31.2832) centre (0, 0) ccw projected
  arc A310 (8.7633, -29.944) -> (9.889, -31.4835) centre (17.9847, -24.3828) ccw projected
  arc A311 (8.1737, -30.1103) -> (8.7633, -29.944) centre (0, 0) ccw projected
  arc A312 (8.0183, -32.011) -> (8.1737, -30.1103) centre (-2.5945, -30.1867) ccw projected
  arc A313 (7.3883, -32.1623) -> (8.0183, -32.011) centre (0, 0) ccw projected
  arc A314 (6.3869, -30.5393) -> (7.3883, -32.1623) centre (16.0162, -25.7187) ccw projected
  arc A315 (5.7861, -30.6588) -> (6.3869, -30.5393) centre (0, 0) ccw projected
  arc A316 (5.4821, -32.5415) -> (5.7861, -30.6588) centre (-4.9549, -29.8901) ccw projected
  arc A317 (4.8421, -32.6428) -> (5.4821, -32.5415) centre (0, 0) ccw projected
  arc A318 (3.9712, -30.9462) -> (4.8421, -32.6428) centre (13.9489, -26.896) ccw projected
  arc A319 (3.3628, -31.0182) -> (3.9712, -30.9462) centre (0, 0) ccw projected
  circle A320 centre (0, 0) radius 36.3 projected
  circle A321 centre (0, 0) radius 33
  point P0 (-32.9221, -2.2661)
  point P1 (-32.9984, -0.324)
  point P2 (-32.9984, 0.324)
  point P3 (-32.9221, 2.2661)
  point P4 (-32.8713, 2.912)
  point P5 (-32.6428, 4.8421)
  point P6 (-32.5415, 5.4821)
  point P7 (-32.1623, 7.3883)
  point P8 (-32.011, 8.0183)
  point P9 (-31.4835, 9.889)
  point P10 (-31.2832, 10.5052)
  point P11 (-30.3626, 12.9273)
  point P12 (-29.5489, 14.6923)
  point P13 (-29.2547, 15.2696)
  point P14 (-28.305, 16.9654)
  point P15 (-27.9665, 17.5179)
  point P16 (-26.5058, 19.6581)
  point P17 (-24.8818, 21.6771)
  point P18 (-23.5625, 23.1043)
  point P19 (-23.1043, 23.5625)
  point P20 (-21.6771, 24.8818)
  point P21 (-21.1844, 25.3026)
  point P22 (-19.6581, 26.5058)
  point P23 (-19.1339, 26.8867)
  point P24 (-16.9654, 28.305)
  point P25 (-15.2696, 29.2547)
  point P26 (-14.6923, 29.5489)
  point P27 (-12.3286, 30.6105)
  point P28 (-7.3883, 32.1623)
  point P29 (-5.4821, 32.5415)
  point P30 (-4.8421, 32.6428)
  point P31 (-2.912, 32.8713)
  point P32 (-2.2661, 32.9221)
  point P33 (-0.324, 32.9984)
  point P34 (0.324, 32.9984)
  point P35 (2.2661, 32.9221)
  point P36 (2.912, 32.8713)
  point P37 (4.8421, 32.6428)
  point P38 (7.3883, 32.1623)
  point P39 (8.0183, 32.011)
  point P40 (9.889, 31.4835)
  point P41 (10.5052, 31.2832)
  point P42 (12.9273, 30.3626)
  point P43 (14.6923, 29.5489)
  point P44 (15.2696, 29.2547)
  point P45 (16.9654, 28.305)
  point P46 (17.5179, 27.9665)
  point P47 (19.1339, 26.8867)
  point P48 (19.6581, 26.5058)
  point P49 (21.6771, 24.8818)
  point P50 (23.5625, 23.1043)
  point P51 (25.3026, 21.1844)
  point P52 (26.8867, 19.1339)
  point P53 (27.9665, 17.5179)
  point P54 (28.305, 16.9654)
  point P55 (29.2547, 15.2696)
  point P56 (29.5489, 14.6923)
  point P57 (30.3626, 12.9273)
  point P58 (30.6105, 12.3286)
  point P59 (31.2832, 10.5052)
  point P60 (32.011, 8.0183)
  point P61 (32.1623, 7.3883)
  point P62 (32.5415, 5.4821)
  point P63 (32.6428, 4.8421)
  point P64 (32.8713, 2.912)
  point P65 (32.9984, 0.324)
  point P66 (32.9984, -0.324)
  point P67 (32.9221, -2.2661)
  point P68 (32.8713, -2.912)
  point P69 (32.6428, -4.8421)
  point P70 (32.5415, -5.4821)
  point P71 (32.1623, -7.3883)
  point P72 (32.011, -8.0183)
  point P73 (31.4835, -9.889)
  point P74 (31.2832, -10.5052)
  point P75 (30.3626, -12.9273)
  point P76 (29.5489, -14.6923)
  point P77 (29.2547, -15.2696)
  point P78 (26.8867, -19.1339)
  point P79 (26.5058, -19.6581)
  point P80 (24.8818, -21.6771)
  point P81 (23.5625, -23.1043)
  point P82 (23.1043, -23.5625)
  point P83 (21.1844, -25.3026)
  point P84 (19.6581, -26.5058)
  point P85 (19.1339, -26.8867)
  point P86 (16.9654, -28.305)
  point P87 (15.2696, -29.2547)
  point P88 (12.3286, -30.6105)
  point P89 (10.5052, -31.2832)
  point P90 (9.889, -31.4835)
  point P91 (7.3883, -32.1623)
  point P92 (5.4821, -32.5415)
  point P93 (4.8421, -32.6428)
  point P94 (2.912, -32.8713)
  point P95 (2.2661, -32.9221)
  point P96 (-0.324, -32.9984)
  point P97 (-2.2661, -32.9221)
  point P98 (-2.912, -32.8713)
  point P99 (-4.8421, -32.6428)
  point P100 (-5.4821, -32.5415)
  point P101 (-7.3883, -32.1623)
  point P102 (-9.889, -31.4835)
  point P103 (-10.5052, -31.2832)
  point P104 (-12.3286, -30.6105)
  point P105 (-12.9273, -30.3626)
  point P106 (-14.6923, -29.5489)
  point P107 (-15.2696, -29.2547)
  point P108 (-16.9654, -28.305)
  point P109 (-17.5179, -27.9665)
  point P110 (-19.1339, -26.8867)
  point P111 (-19.6581, -26.5058)
  point P112 (-21.1844, -25.3026)
  point P113 (-21.6771, -24.8818)
  point P114 (-23.1043, -23.5625)
  point P115 (-23.5625, -23.1043)
  point P116 (-24.8818, -21.6771)
  point P117 (-25.3026, -21.1844)
  point P118 (-26.5058, -19.6581)
  point P119 (-26.8867, -19.1339)
  point P120 (-28.305, -16.9654)
  point P121 (-29.2547, -15.2696)
  point P122 (-29.5489, -14.6923)
  point P123 (-30.6105, -12.3286)
  point P124 (-31.2832, -10.5052)
  point P125 (-31.4835, -9.889)
  point P126 (-32.011, -8.0183)
  point P127 (-32.1623, -7.3883)
  point P128 (-32.5415, -5.4821)
  point P129 (-32.6428, -4.8421)
  point P130 (-32.8713, -2.912)
  constraints: 1 coincident, 2 other
extrude "Extrusion2" add sketch "Sketch3" along normal blind 2
sketch "Sketch4" plane through (0, 0, 7) normal (0, 0, 1) x (1, 0, 0)
  circle A0 centre (0, 0) radius 34
  circle A1 centre (0, 0) radius 32
  dimension "d55" = 68
  dimension "d56" = 64
  constraints: 2 centre point, 2 coincident
  measures "d55" diameter of A0
  measures "d56" diameter of A1
extrude "Extrusion3" add sketch "Sketch4" along normal blind 4
mirror "Mirror1" about plane through (0, 0, 0) normal (0, 0, 1) of "Extrusion3", "Extrusion2"
equation "\"d0\" = 1.1 * da_df"
equation "\"d1\" = da_b"
equation "\"d3\" = da_d"
equation "\"d16\" = da_aw"
equation "\"d47\" = da_aw"
equation "\"d52\" = da_aw"
equation "\"da_df\" = 66"
equation "\"da_b\" = 10"
equation "\"da_d\" = 64"
equation "\"da_aw\" = 24"
body "Solid1"
body "Srf1"
